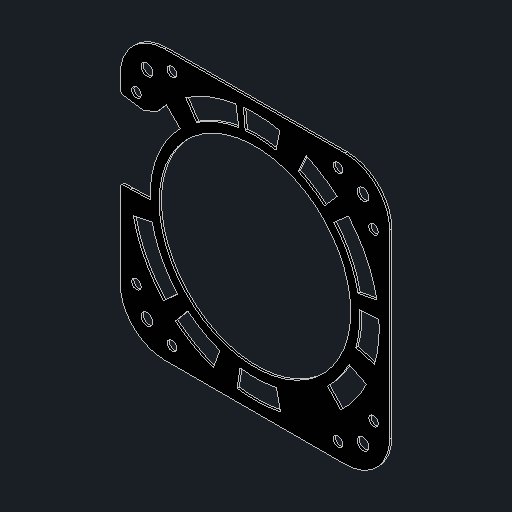
# Autodesk Inventor part: stator_mount_02_p
Saved by Autodesk Inventor 2026.1 (Build 301233000, 233)
## iProperties
Created: 2026-04-12
Part Number: stator_mount_02_p
Material: PC/ABS Plastic
Document SubType Name: Modeling
Designer: aaron
Density: 1.1 g/cm^3
Appearance: Smooth - White
Author: aaron
Autodesk Inventor part; units mm, degrees
ref_plane "YZ Plane" through (0, 0, 0) normal (1, 0, 0) x (0, 1, 0)
ref_plane "XZ Plane" through (0, 0, 0) normal (0, 1, 0) x (-1, 0, 0)
ref_plane "XY Plane" through (0, 0, 0) normal (0, 0, 1) x (1, 0, 0)
sketch "Sketch1" plane through (0, 0, 0) normal (0, 0, 1) x (1, 0, 0)
  circle A0 centre (0, 0) radius 29
  circle A1 centre (0, 0) radius 60.5
  line L0 (-40.5, 60.5) -> (40.5, 60.5)
  line L1 (60.5, 40.5) -> (60.5, -40.5)
  line L2 (40.5, -60.5) -> (-40.5, -60.5)
  line L3 (-60.5, -40.5) -> (-60.5, 40.5)
  arc A2 (-40.5, 60.5) -> (-60.5, 40.5) centre (-40.5, 40.5) ccw
  arc A3 (60.5, 40.5) -> (40.5, 60.5) centre (40.5, 40.5) ccw
  arc A4 (40.5, -60.5) -> (60.5, -40.5) centre (40.5, -40.5) ccw
  arc A5 (-60.5, -40.5) -> (-40.5, -60.5) centre (-40.5, -40.5) ccw
  dimension "d0" = 58
  dimension "d1" = 121
  dimension "d2" = 20
  constraints: 12 tangent, 8 end point, 8 point on circle, 6 centre point, 3 equal radius, 2 coincident, 2 parallel, 1 horizontal, 1 perpendicular
  measures "d0" diameter of A0
  measures "d1" diameter of A1
  measures "d2" radius of A2
extrude "Extrusion1" add sketch "Sketch1" along normal blind 1
sketch "Sketch2" plane through (0, 0, 1) normal (0, 0, 1) x (1, 0, 0)
  circle A0 centre (0.027076, 0) radius 29
  line L0 (9.676425, -46.097047) -> (11.455129, -54.594307)
  arc A1 (-7.962925, -55.202343) -> (11.455129, -54.594307) centre (0.027076, 0) ccw
  line L1 (-7.962925, -55.202343) -> (-6.719332, -46.610446)
  arc A2 (-6.719332, -46.610446) -> (9.676425, -46.097047) centre (0.027076, 0) ccw
  line L2 (-26.22683, 39.099618) -> (-31.066321, 46.307013)
  arc A3 (-8.564139, 55.111975) -> (-31.066321, 46.307013) centre (0.027076, 0) ccw
  line L3 (-8.564139, 55.111975) -> (-7.226971, 46.534143)
  arc A4 (-7.226971, 46.534143) -> (-26.22683, 39.099618) centre (0.027076, 0) ccw
  line L4 (53.725945, -15.085432) -> (45.368054, -12.737479)
  arc A5 (45.368054, -12.737479) -> (47.037995, 2.832164) centre (0.027076, 0) ccw
  line L5 (47.037995, 2.832164) -> (55.703713, 3.354229)
  arc A6 (53.725945, -15.085432) -> (55.703713, 3.354229) centre (0.027076, 0) ccw
  line L6 (54.804414, 10.515798) -> (46.278666, 8.87908)
  arc A7 (46.278666, 8.87908) -> (35.452755, 31.033352) centre (0.027076, 0) ccw
  line L7 (35.452755, 31.033352) -> (41.982918, 36.753858)
  arc A8 (54.804414, 10.515798) -> (41.982918, 36.753858) centre (0.027076, 0) ccw
  line L8 (-15.75806, -44.372032) -> (-18.6678, -52.551313)
  arc A9 (-35.68795, -42.84362) -> (-18.6678, -52.551313) centre (0.027076, 0) ccw
  line L9 (-35.68795, -42.84362) -> (-30.129131, -36.17528)
  arc A10 (-30.129131, -36.17528) -> (-15.75806, -44.372032) centre (0.027076, 0) ccw
  line L10 (11.249897, 54.636866) -> (9.503135, 46.132982)
  arc A11 (9.503135, 46.132982) -> (-4.364808, 46.890927) centre (0.027076, 0) ccw
  line L11 (-4.364808, 46.890927) -> (-5.174383, 55.534527)
  arc A12 (11.249897, 54.636866) -> (-5.174383, 55.534527) centre (0.027076, 0) ccw
  line L12 (38.573882, -40.314793) -> (32.574314, -34.040049)
  arc A13 (32.574314, -34.040049) -> (42.287253, -20.787618) centre (0.027076, 0) ccw
  line L13 (42.287253, -20.787618) -> (50.077248, -24.619486)
  arc A14 (38.573882, -40.314793) -> (50.077248, -24.619486) centre (0.027076, 0) ccw
  line L14 (36.918402, 41.83502) -> (31.176499, 35.323662)
  arc A15 (31.176499, 35.323662) -> (19.464033, 42.898163) centre (0.027076, 0) ccw
  line L15 (19.464033, 42.898163) -> (23.046928, 50.80576)
  arc A16 (36.918402, 41.83502) -> (23.046928, 50.80576) centre (0.027076, 0) ccw
  line L16 (-34.657821, -31.859153) -> (-41.051432, -37.731883)
  arc A17 (-54.567232, -11.428054) -> (-41.051432, -37.731883) centre (0.027076, 0) ccw
  line L17 (-54.567232, -11.428054) -> (-46.069972, -9.649349)
  arc A18 (-46.069972, -9.649349) -> (-34.657821, -31.859153) centre (0.027076, 0) ccw
  circle A19 centre (37.302278, 53.24997) radius 2.15
  circle A20 centre (16.523176, 28.58109) radius 1.25
  circle A21 centre (-37.248127, -53.24997) radius 2.15
  circle A22 centre (-37.262658, 53.239795) radius 2.15
  circle A23 centre (48.533694, -48.493381) radius 2.65
  circle A24 centre (-48.466306, -48.506618) radius 2.65
  circle A25 centre (-53.222894, 37.275202) radius 2.15
  circle A26 centre (-53.212719, -37.289734) radius 2.15
  circle A27 centre (16.530975, -28.576586) radius 1.25
  circle A28 centre (53.26687, 37.289734) radius 2.15
  circle A29 centre (53.277046, -37.275202) radius 2.15
  circle A30 centre (-16.469024, -28.58109) radius 1.25
  circle A31 centre (-16.476824, 28.576586) radius 1.25
  circle A32 centre (48.520457, 48.506618) radius 2.65
  circle A33 centre (-48.479542, 48.493381) radius 2.65
  circle A34 centre (-32.972924, -0.004503) radius 1.25
  circle A35 centre (37.316809, -53.239795) radius 2.15
  circle A36 centre (33.027075, 0.004503) radius 1.25
  line L18 (-59.489133, 33.281523) -> (-60.477624, 34.433691)
  line L19 (-59.489133, 33.281523) -> (-50.139097, 31.841989)
  line L20 (-43.828439, 34.464948) -> (-50.139097, 31.841989)
  arc A37 (-39.727407, 39.124416) -> (-43.828439, 34.464948) centre (0.027076, 0) ccw
  line L21 (-39.727407, 39.124416) -> (-33.539872, 33.034947)
  arc A38 (-33.539872, 33.034947) -> (-47.048538, -1.390807) centre (0.027076, 0) ccw
  line L22 (-47.048538, -1.390807) -> (-55.726181, -1.647181)
  line L23 (-55.726181, -1.647181) -> (-59.4727, -1.647692)
  line L24 (-60.472564, -2.647828) -> (-59.4727, -1.647692)
  line L25 (-60.472564, -2.647828) -> (-60.467398, -40.499996)
  arc A39 (-60.5, -40.5) -> (-40.464668, -60.505526) centre (-40.467397, -40.505526) ccw
  line L26 (-40.464668, -60.505526) -> (40.535331, -60.494473)
  arc A40 (40.535331, -60.494473) -> (60.532602, -40.491744) centre (40.532602, -40.494473) ccw
  line L27 (60.532602, -40.491744) -> (60.521548, 40.508256)
  arc A41 (60.521548, 40.508256) -> (40.518819, 60.505526) centre (40.521549, 40.505526) ccw
  line L28 (40.518819, 60.505526) -> (-40.48118, 60.494473)
  arc A42 (-40.48118, 60.494473) -> (-60.478451, 40.491744) centre (-40.478451, 40.494473) ccw
  line L29 (-60.478452, 40.500003) -> (-60.477624, 34.433691)
  line L30 (-60.5, 40.5) -> (-60.5, -40.5)
  circle A43 centre (0.027076, 0) radius 43
  point P0 (0, 0)
  point P1 (-60.5, 34.441709)
  point P2 (-60.5, -2.639369)
  constraints: 2 other
sketch "Sketch2 outline for Extrusion2" plane through (0, 0, 1) normal (0, 0, 1) x (1, 0, 0)
  circle A0 centre (37.302278, 53.24997) radius 2.15
  circle A1 centre (-37.262658, 53.239795) radius 2.15
  circle A2 centre (-53.222894, 37.275202) radius 2.15
  circle A3 centre (-48.479542, 48.493381) radius 2.65
  arc A4 (-7.962925, -55.202343) -> (11.455129, -54.594307) centre (0.027076, 0) ccw
  line L0 (-6.719332, -46.610446) -> (-7.962925, -55.202343)
  arc A5 (9.676425, -46.097047) -> (-6.719332, -46.610446) centre (0.027076, 0) cw
  line L1 (11.455129, -54.594307) -> (9.676425, -46.097047)
  circle A6 centre (37.316809, -53.239795) radius 2.15
  circle A7 centre (53.277046, -37.275202) radius 2.15
  circle A8 centre (48.533694, -48.493381) radius 2.65
  arc A9 (38.573882, -40.314793) -> (50.077248, -24.619486) centre (0.027076, 0) ccw
  line L2 (32.574314, -34.040049) -> (38.573882, -40.314793)
  arc A10 (42.287253, -20.787618) -> (32.574314, -34.040049) centre (0.027076, 0) cw
  line L3 (50.077248, -24.619486) -> (42.287253, -20.787618)
  circle A11 centre (53.26687, 37.289734) radius 2.15
  circle A12 centre (48.520457, 48.506618) radius 2.65
  arc A13 (53.725945, -15.085432) -> (55.703713, 3.354229) centre (0.027076, 0) ccw
  line L4 (45.368054, -12.737479) -> (53.725945, -15.085432)
  arc A14 (47.037995, 2.832164) -> (45.368054, -12.737479) centre (0.027076, 0) cw
  line L5 (55.703713, 3.354229) -> (47.037995, 2.832164)
  arc A15 (54.804414, 10.515798) -> (41.982918, 36.753858) centre (0.027076, 0) ccw
  line L6 (46.278666, 8.87908) -> (54.804414, 10.515798)
  arc A16 (35.452755, 31.033352) -> (46.278666, 8.87908) centre (0.027076, 0) cw
  line L7 (41.982918, 36.753858) -> (35.452755, 31.033352)
  arc A17 (36.918402, 41.83502) -> (23.046928, 50.80576) centre (0.027076, 0) ccw
  line L8 (31.176499, 35.323662) -> (36.918402, 41.83502)
  arc A18 (19.464033, 42.898163) -> (31.176499, 35.323662) centre (0.027076, 0) cw
  line L9 (23.046928, 50.80576) -> (19.464033, 42.898163)
  arc A19 (11.249897, 54.636866) -> (-5.174383, 55.534527) centre (0.027076, 0) ccw
  line L10 (9.503135, 46.132982) -> (11.249897, 54.636866)
  arc A20 (-4.364808, 46.890927) -> (9.503135, 46.132982) centre (0.027076, 0) cw
  line L11 (-5.174383, 55.534527) -> (-4.364808, 46.890927)
  arc A21 (-8.564139, 55.111975) -> (-31.066321, 46.307013) centre (0.027076, 0) ccw
  line L12 (-7.226971, 46.534143) -> (-8.564139, 55.111975)
  arc A22 (-26.22683, 39.099618) -> (-7.226971, 46.534143) centre (0.027076, 0) cw
  line L13 (-31.066321, 46.307013) -> (-26.22683, 39.099618)
  circle A23 centre (0.027076, 0) radius 43
  circle A24 centre (-37.248127, -53.24997) radius 2.15
  arc A25 (-35.68795, -42.84362) -> (-18.6678, -52.551313) centre (0.027076, 0) ccw
  line L14 (-30.129131, -36.17528) -> (-35.68795, -42.84362)
  arc A26 (-15.75806, -44.372032) -> (-30.129131, -36.17528) centre (0.027076, 0) cw
  line L15 (-18.6678, -52.551313) -> (-15.75806, -44.372032)
  circle A27 centre (-48.466306, -48.506618) radius 2.65
  circle A28 centre (-53.212719, -37.289734) radius 2.15
  arc A29 (-54.567232, -11.428054) -> (-41.051432, -37.731883) centre (0.027076, 0) ccw
  line L16 (-46.069972, -9.649349) -> (-54.567232, -11.428054)
  arc A30 (-34.657821, -31.859153) -> (-46.069972, -9.649349) centre (0.027076, 0) cw
  line L17 (-41.051432, -37.731883) -> (-34.657821, -31.859153)
  line L18 (-60.472564, -2.647828) -> (-59.4727, -1.647692)
  line L19 (-60.5, -40.5) -> (-60.472564, -2.647828)
  line L20 (-60.5, 40.5) -> (-60.5, -40.5)
  line L21 (-60.477624, 34.433691) -> (-60.5, 40.5)
  line L22 (-59.489133, 33.281523) -> (-60.477624, 34.433691)
  line L23 (-50.139097, 31.841989) -> (-59.489133, 33.281523)
  line L24 (-43.828439, 34.464948) -> (-50.139097, 31.841989)
  arc A31 (-39.727407, 39.124416) -> (-43.828439, 34.464948) centre (0.027076, 0) ccw
  line L25 (-33.539872, 33.034947) -> (-39.727407, 39.124416)
  arc A32 (-47.048538, -1.390807) -> (-33.539872, 33.034947) centre (0.027076, 0) cw
  line L26 (-55.726181, -1.647181) -> (-47.048538, -1.390807)
  line L27 (-59.4727, -1.647692) -> (-55.726181, -1.647181)
extrude "Extrusion2" cut sketch "Sketch2 outline for Extrusion2" against normal through all
body "Solid1"
